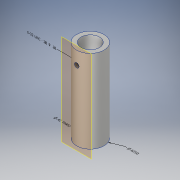
# Autodesk Inventor part: ToolHolderAdapter_v2
Saved by Autodesk Inventor 2018.3 (Build 223284000, 284)
## iProperties
Created: 2019-09-24
Part Number: ToolHolderAdapter_v2
Material: Aluminum 6061
Document SubType Name: Modeling
Designer: sshanbhag
Density: 2.7 g/cm^3
Appearance: Aluminum - Flat
Author: sshanbhag
Autodesk Inventor part; units mm, degrees
ref_plane "YZ Plane" through (0, 0, 0) normal (1, 0, 0) x (0, 1, 0)
ref_plane "XZ Plane" through (0, 0, 0) normal (0, 1, 0) x (-1, 0, 0)
sketch "Sketch1" plane through (0, 0, 0) normal (0, 1, 0) x (-1, 0, 0)
  circle A0 centre (0, 0) radius 7.9375
  dimension "d35" = 15.875
  constraints: 1 centre point, 1 coincident
  measures "d35" diameter of A0
extrude "Extrusion1" add sketch "Sketch1" along normal blind 48.26
hole "Hole1" at (0, 0, 0) direction (0, 1, 0) diameter 10.668 end through all
ref_plane "Work Plane1" through (0, 0, 7.9375) normal (0, 0, 1) x (1, 0, 0)
sketch "Sketch2" plane through (0, 0, 7.9375) normal (0, 0, 1) x (1, 0, 0)
  line L0 (-7.9375, 0) -> (-7.9375, 48.26) projected
  line L1 (-7.9375, 0) -> (7.9375, 0) projected
  line L2 (7.9375, 48.26) -> (-7.9375, 48.26) projected
  point P0 (0, 0)
  point P1 (0, 40.64)
  dimension "d11" = 40.64
  dimension "d42" = 7.62
  constraints: 1 vertical alignment
  measures "d11" distance from line of L1 point (0, 40.64)
  measures "d42" distance from line of L2 point (0, 40.64)
hole "Hole2" at (0, 40.64, 7.9375) direction (0, 0, -1) diameter 2.6416 depth 10.16 tip angle 118 thread size "6-32 UNC" class "2B" standard "ANSI Unified Screw Threads"
body "Solid1"
